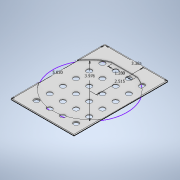
# Autodesk Inventor part: 100mm wafer wellplate - corral mask - with flat - lowdensity
Saved by Autodesk Inventor 2020 (Build 240168000, 168)
## iProperties
Created: 2022-04-03
Part Number: 100mm wafer wellplate - corral mask - with flat - lowdensity
Material: Generic
Document SubType Name: Modeling
Designer: Beaucage
Density: 1 g/cm^3
Appearance: Default
Author: Beaucage
Autodesk Inventor part; units mm, degrees
ref_plane "YZ Plane" through (0, 0, 0) normal (1, 0, 0) x (0, 1, 0)
ref_plane "XZ Plane" through (0, 0, 0) normal (0, 1, 0) x (-1, 0, 0)
ref_plane "XY Plane" through (0, 0, 0) normal (0, 0, 1) x (1, 0, 0)
sketch "Sketch1" plane through (0, 0, 0) normal (0, 1, 0) x (-1, 0, 0)
  line L0 (0, 0) -> (85.48, 0)
  line L1 (85.48, 0) -> (85.48, -127.76)
  line L2 (85.48, -127.76) -> (0, -127.76)
  line L3 (0, -127.76) -> (0, 0)
  line L4 (42.74, -127.76) -> (42.74, -63.879)
  circle A0 centre (42.1561, -63.879) radius 50.5
  line L5 (26.485, -111.163) -> (58.985, -111.1664)
  line L6 (42.74, -63.879) -> (42.7347, -113.879)
  line L7 (26.485, -111.163) -> (24.4227, -111.163)
  line L8 (58.985, -111.1664) -> (59.8896, -111.163)
  point P0 (85.48, -37.9311)
  point P1 (85.48, -89.8269)
  point P2 (0, -91.6839)
  point P3 (0, -36.0741)
  point P4 (42.735, -111.1647)
  point P5 (42.74, -111.1647)
  point P6 (42.74, -114.3756)
  dimension "d0" = 85.48
  dimension "d1" = 127.76
  dimension "d2" = 63.881
  dimension "d3" = 101
  dimension "d4" = 32.5
  constraints: 18 end point, 4 point on circle, 3 perpendicular, 3 point on line, 2 horizontal, 2 parallel, 1 centre point, 1 coincident, 1 midpoint
  measures "d0" distance of L1.end L2.end
  measures "d1" distance of L0.end L1.end
  measures "d2" distance of L4.start L4.end
  measures "d3" diameter of A0
  measures "d4" distance of L5.start L5.end
extrude "Extrusion1" add sketch "Sketch1" along normal blind 1.7938 contours L0 L1 A0 L3 | A0 L4 L2 L3 | L1 L2 L4 A0 | L7 L5 L4 A0 | A0 L4 L5 L8
extrude "Extrusion2" add sketch "Sketch1" along normal blind 0.7937 contours A0 L1 L8 L5 L4 L6 L7 L3 | L7 L5 L4 A0 | A0 L4 L5 L8 | L5 L6 L4
sketch "Sketch2" plane through (0, 1.7938, 0) normal (0, 1, 0) x (1, 0, 0)
  line L0 (-85.48, 127.76) -> (-85.48, 0) projected
  line L1 (-85.48, 25.2748) -> (-79.48, 25.2748)
  line L2 (-85.48, 25.2748) -> (-79.48, 25.2748) construction
  arc A0 (-85.48, 37.9311) -> (0, 36.0741) centre (-42.1561, 63.879) ccw projected
  line L3 (-42.1561, 13.379) -> (-42.1561, 19.379)
  line L4 (-42.1561, 19.379) -> (-85.48, 19.379)
  line L5 (-85.48, 19.379) -> (-79.48, 19.379)
  line L6 (0, 0) -> (0, 14.38)
  line L7 (0, 0) -> (0, 127.76) projected
  line L8 (0, 14.38) -> (-11.34, 14.38)
  dimension "d9" = 6
  dimension "d10" = 0
  dimension "d24" = 6
  dimension "d25" = 6
  dimension "d26" = 14.38
  dimension "d27" = 11.34
  constraints: 14 end point, 4 point on line, 3 perpendicular, 1 collinear, 1 horizontal, 1 point on circle, 1 vertical
  measures "d9" distance of L1.start L1.end
  measures "d10" distance between parallel lines of L1 L2
  measures "d24" distance of L3.start L3.end
  measures "d25" distance of L4.end L5.end
  measures "d26" distance of L6.start L6.end
  measures "d27" distance of L6.end L8.end
hole "Hole1" at (-11.34, 1.7938, -14.38) direction (0, -1, 0) diameter 7 end through all
pattern_linear "Rectangular Pattern1" count 6 spacing 18 along (0, 0, -1) count 4 spacing 18 along (-1, 0, 0) of "Hole1"
body "Solid1"
